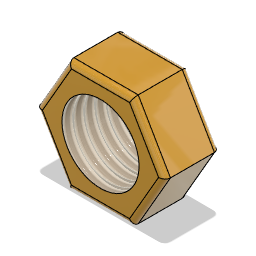
Ecrous M16 (Autodesk Fusion 360 design; units mm, degrees)
Autodesk Fusion 360 part; units mm, degrees
sketch "Sketch1" plane through (0, 0, 0) normal (0, 0, 1) x (1, 0, 0)
  circle A0 centre (0, 0) radius 8.15
  circle A1 centre (0, 0) radius 9.15 construction
  circle A2 centre (0, 0) radius 10.15 construction
  line L0 (-5.8601, 10.15) -> (-11.7202, 0)
  line L1 (-11.7202, 0) -> (-5.8601, -10.15)
  line L2 (-5.8601, -10.15) -> (5.8601, -10.15)
  line L3 (5.8601, -10.15) -> (11.7202, 0)
  line L4 (11.7202, 0) -> (5.8601, 10.15)
  line L5 (5.8601, 10.15) -> (-5.8601, 10.15)
  dimension "d1" = 16.3
  dimension "d2" = 1
  dimension "d3" = 2
  constraint coincident A0.centre A1.centre
  measures "d1" diameter of A0
extrude "Extrude1" add sketch "Sketch1" along normal blind 10
fillet "Fillet1" radius 1 6 edges at (-8.7902, 5.075, 10) (-8.7902, -5.075, 10) (0, -10.15, 10) (8.7902, -5.075, 10) (8.7902, 5.075, 10) (0, 10.15, 10)
fillet "Fillet2" radius 1 6 edges at (0, 10.15, 0) (8.7902, 5.075, 0) (8.7902, -5.075, 0) (0, -10.15, 0) (-8.7902, -5.075, 0) (-8.7902, 5.075, 0)
thread "Thread1" "ISO Metric profile 16.0 M16x2 6H" major diameter 16.2505 minor diameter 14.0225 pitch 2 angle 60 resizes the face on face at (8.1399, -0.4062, 6.6667)
